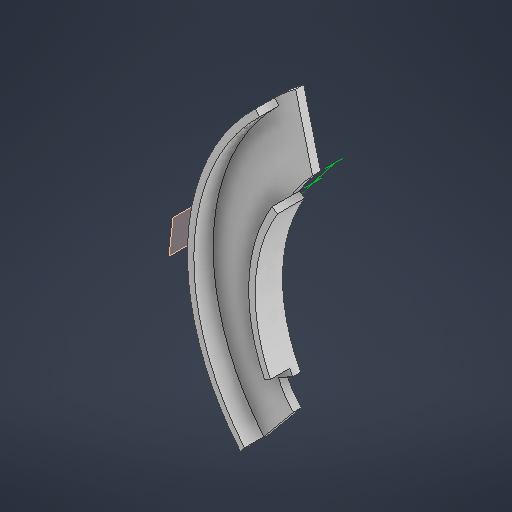
# Autodesk Inventor part: outside33
Saved by Autodesk Inventor 2026.2 (Build 302298000, 298)
## iProperties
Created: 2026-03-14
Part Number: outside33
Material: Generic
Document SubType Name: Modeling
Designer: danda
Density: 1 g/cm^3
Appearance: Default
Author: danda
Autodesk Inventor part; units mm, degrees
ref_plane "YZ Plane" through (0, 0, 0) normal (1, 0, 0) x (0, 1, 0)
ref_plane "XZ Plane" through (0, 0, 0) normal (0, 1, 0) x (-1, 0, 0)
ref_plane "XY Plane" through (0, 0, 0) normal (0, 0, 1) x (1, 0, 0)
sketch "Sketch1" plane through (0, 0, 0) normal (0, 0, 1) x (1, 0, 0)
  arc A0 (967.6192, 924.0732) -> (967.7873, 1075.2272) centre (902.2196, 999.723) ccw
  arc A1 (983.2683, 893.0126) -> (983.4428, 1106.3006) centre (902.2196, 999.723) ccw
  line L0 (965.7611, 927.7614) -> (985.0977, 889.3816)
  line L1 (966.6908, 925.9161) -> (1011.6908, 925.9161) construction
  arc A2 (985.0977, 889.3816) -> (985.2727, 1109.9327) centre (902.2196, 999.723) ccw
  line L2 (965.9281, 1071.5369) -> (985.2727, 1109.9327)
  arc A3 (965.7611, 927.7614) -> (965.9281, 1071.5369) centre (902.2196, 999.723) ccw
  line L3 (977.4986, 940.149) -> (980.6353, 937.6667)
  point P0 (0, 0)
  point P1 (983.9681, 893.1)
  point P2 (990.6031, 1100.4422)
  point P3 (968.1775, 1074.8866)
  dimension "d28" = 100
  dimension "d33" = 63.26
  dimension "d34" = 4
  dimension "d40" = 4
  dimension "d41" = 4
  constraints: 10 point on circle, 8 end point, 5 point on line, 4 centre point, 1 horizontal
  measures "d28" radius of A0
  measures "d33" angle of L0 L1
  measures "d34" radial gap between concentric circles of A1 A2
  measures "d40" radial gap between concentric circles of A0 A3
  measures "d41" distance of L3.start L3.end
extrude "Extrusion6" add sketch "Sketch1" along normal blind 5
extrude "Extrusion7" add sketch "Sketch1" along normal blind 17 contours L3 A3 L2 A0 | A1 L2 A2 L0
sketch "Sketch5" plane through (0, 0, 5) normal (0, 0, 1) x (1, 0, 0)
  arc A0 (965.7611, 927.7614) -> (977.4986, 940.149) centre (902.2196, 999.723) ccw projected
  line L0 (965.7611, 927.7614) -> (970.2605, 918.8308)
  line L1 (965.7611, 927.7614) -> (983.2683, 893.0126) projected
  line L2 (977.4986, 940.149) -> (985.1361, 933.6938)
  arc A1 (965.7611, 927.7614) -> (977.4986, 940.149) centre (902.2196, 999.723) ccw
  arc A2 (965.7611, 927.7614) -> (974.9009, 937.006) centre (902.2196, 999.723) ccw
  line L3 (974.9009, 937.006) -> (982.5384, 930.5509)
  arc A3 (970.2605, 918.8308) -> (982.5384, 930.5509) centre (950.8165, 951.4915) ccw
  point P0 (0, 0)
  dimension "d42" = 10
  dimension "d43" = 10
  dimension "d46" = 13
  dimension "d47" = 10
  constraints: 7 point on circle, 6 end point, 3 centre point, 1 concentric, 1 parallel, 1 point on line
  measures "d42" distance of L0.start L0.end
  measures "d43" distance of L2.start L2.end
  measures "d46" distance of L0.start L3.start
  measures "d47" distance of L3.start L3.end
extrude "Extrusion8" cut sketch "Sketch5" along normal through all both and the other way through all
sketch "Sketch6" plane through (0, 0, 5) normal (0, 0, 1) x (1, 0, 0)
  arc A0 (974.9009, 937.006) -> (965.9281, 1071.5369) centre (902.2196, 999.723) ccw projected
  arc A1 (985.0977, 889.3816) -> (985.2727, 1109.9327) centre (902.2196, 999.723) ccw projected
  line L0 (985.8441, 1046.8712) -> (1027.8759, 1046.8712) construction
  line L1 (985.2727, 1109.9327) -> (965.9281, 1071.5369) projected
  line L2 (965.9281, 1071.5369) -> (985.2727, 1109.9327)
  arc A2 (985.8441, 1046.8712) -> (965.9281, 1071.5369) centre (902.2196, 999.723) ccw
  arc A3 (1007.3627, 1089.1038) -> (985.2727, 1109.9327) centre (902.2196, 999.723) ccw
  line L3 (985.8441, 1046.8712) -> (1007.3627, 1089.1038)
  point P0 (0, 0)
  dimension "d51" = 63
  constraints: 6 end point, 6 point on circle, 2 centre point, 2 concentric, 1 collinear, 1 horizontal
  measures "d51" angle of L3 L0
extrude "Extrusion9" cut sketch "Sketch6" along normal through all both and the other way through all
ref_plane "Work Plane1" through (1039.37, 984.4335, 17) normal (0.9938434, -0.1107936, 0) x (0.1107936, 0.9938434, 0)
mirror "Mirror1" about plane through (1039.37, 984.4335, 17) normal (0.9938434, -0.1107936, 0) remove original yes
sketch "Sketch7" plane through (1176.5204, 969.144, 5) normal (0, 0, 1) x (0.9942316, -0.1072545, 0)
  line L0 (-84.9964, -52.684) -> (-81.5966, -50.5766) projected
  arc A0 (-77.6856, 56.3999) -> (-81.5966, -50.5766) centre (0, 0) ccw
  arc A1 (-80.9225, 58.7499) -> (-87.0358, -49.242) centre (0, 0) ccw
  line L1 (-87.0358, -49.242) -> (-87.1038, -49.2841)
  line L2 (-79.3475, 60.8603) -> (-77.6856, 56.3999) projected
  line L3 (-77.6856, 56.3999) -> (-79.3475, 60.8603)
  line L4 (-79.3475, 60.8603) -> (-77.6856, 56.3999)
  line L5 (-87.0358, 40.5064) -> (-90.5829, 42.3644)
  arc A2 (-79.3475, 60.8603) -> (-84.9964, -52.684) centre (0, 0) ccw projected
  point P0 (-1065.7887, -1089.7407)
  point P1 (-90.5829, 42.3644)
  dimension "d52" = 4
  constraints: 8 end point, 6 point on circle, 2 centre point, 2 collinear, 1 other
  measures "d52" radial gap between concentric circles of A0 A1
extrude "Extrusion10" cut sketch "Sketch7" along normal through all both and the other way through all contours L5 A1 A2 L2 A0
sketch "Sketch8" plane through (1176.5204, 969.144, 17) normal (0, 0, 1) x (0.9938434, -0.1107936, 0)
  arc A0 (-93.0614, 96.4135) -> (-92.3725, -97.0738) centre (0, 0) ccw projected
  arc A1 (-93.0614, 96.4135) -> (-103.254, 85.4085) centre (0, 0) ccw
  line L0 (-94.5929, 100.4797) -> (-93.0614, 96.4135) projected
  line L1 (-93.0614, 96.4135) -> (-94.5929, 100.4797)
  line L2 (-103.254, 85.4085) -> (-106.3362, 87.958)
  arc A2 (-94.5929, 100.4797) -> (-94.5929, -100.4797) centre (0, 0) ccw projected
  arc A3 (-94.5929, 100.4797) -> (-106.3362, 87.958) centre (0, 0) ccw
  point P0 (-1061.9021, -1093.5283)
  dimension "d58" = 15
  dimension "d59" = 4
  dimension "d60" = 138
  constraints: 6 point on circle, 4 end point, 2 centre point, 1 collinear
  measures "d58" distance of L0.end L2.start
  measures "d59" distance of L2.start L2.end
  measures "d60" radius of A3
extrude "Extrusion11" cut sketch "Sketch8" against normal blind 12
body "Solid2"
